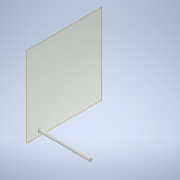
# Autodesk Inventor part: Bar1
Saved by Autodesk Inventor 2021 (Build 250183000, 183)
## iProperties
Created: 2022-07-02
Part Number: Bar1
Material: 一般
Document SubType Name: Modeling
Designer: tazak
Density: 1 g/cm^3
Appearance: 既定
Author: tazak
Autodesk Inventor part; units mm, degrees
ref_plane "XZ Plane" through (0, 0, 0) normal (0, 1, 0) x (-1, 0, 0)
ref_plane "XY Plane" through (0, 0, 0) normal (0, 0, 1) x (1, 0, 0)
ref_plane "作業平面1" through (12000, 0, 0) normal (1, 0, 0) x (0, 1, 0)
sketch "スケッチ13" plane through (12000, 0, 0) normal (1, 0, 0) x (0, 1, 0)
  circle A0 centre (-100, 530) radius 40
  point P0 (0, 0)
  dimension "d84" = 80
  dimension "d85" = 100
  dimension "d86" = 530
  constraints: 1 centre point
  measures "d84" diameter of A0
  measures "d85" horizontal distance of A0.centre point (0, 0)
  measures "d86" vertical distance of point (0, 0) A0.centre
extrude "押し出し12" [suppressed]
sketch "スケッチ14" plane through (12000, 0, 0) normal (1, 0, 0) x (0, 1, 0)
  circle A0 centre (-100, 830) radius 40
  point P0 (0, 0)
  dimension "d89" = 80
  dimension "d90" = 100
  dimension "d91" = 830
  constraints: 1 centre point
  measures "d89" diameter of A0
  measures "d90" horizontal distance of A0.centre point (0, 0)
  measures "d91" vertical distance of point (0, 0) A0.centre
extrude "押し出し13" [suppressed]
sketch "スケッチ15" plane through (12000, 0, 0) normal (1, 0, 0) x (0, 1, 0)
  circle A0 centre (-100, 1130) radius 40
  point P0 (0, 0)
  dimension "d94" = 80
  dimension "d95" = 100
  dimension "d96" = 1130
  constraints: 1 centre point
  measures "d94" diameter of A0
  measures "d95" horizontal distance of A0.centre point (0, 0)
  measures "d96" vertical distance of point (0, 0) A0.centre
extrude "押し出し14" [suppressed]
sketch "スケッチ16" plane through (12000, 0, 0) normal (1, 0, 0) x (0, 1, 0)
  circle A0 centre (-100, 1430) radius 40
  point P0 (0, 0)
  dimension "d99" = 80
  dimension "d100" = 100
  dimension "d101" = 1430
  constraints: 1 centre point
  measures "d99" diameter of A0
  measures "d100" horizontal distance of A0.centre point (0, 0)
  measures "d101" vertical distance of point (0, 0) A0.centre
extrude "押し出し15" [suppressed]
sketch "スケッチ17" plane through (12000, 0, 0) normal (1, 0, 0) x (0, 1, 0)
  circle A0 centre (-100, 1730) radius 40
  point P0 (0, 0)
  dimension "d104" = 80
  dimension "d105" = 100
  dimension "d106" = 1730
  constraints: 1 centre point
  measures "d104" diameter of A0
  measures "d105" horizontal distance of A0.centre point (0, 0)
  measures "d106" vertical distance of point (0, 0) A0.centre
extrude "押し出し16" add sketch "スケッチ17" along normal blind 1500
